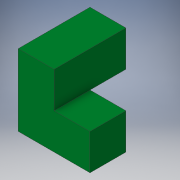
# Autodesk Inventor part: Green part
Saved by Autodesk Inventor 2017 (Build 210142000, 142)
## iProperties
Created: 2016-11-01
Part Number: Green part
Material: Generic
Document SubType Name: Modeling
Designer: rbibb
Density: 1 g/cm^3
Appearance: Default
Author: rbibb
Autodesk Inventor part; units mm, degrees
ref_plane "YZ Plane" through (0, 0, 0) normal (1, 0, 0) x (0, 1, 0)
ref_plane "XZ Plane" through (0, 0, 0) normal (0, 1, 0) x (-1, 0, 0)
ref_plane "XY Plane" through (0, 0, 0) normal (0, 0, 1) x (1, 0, 0)
sketch "Sketch1" plane through (0, 0, 0) normal (1, 0, 0) x (0, 1, 0)
  line L0 (14.195, 33.7604) -> (-4.855, 33.7604)
  line L1 (-4.855, 33.7604) -> (-4.855, -4.3396)
  line L2 (-4.855, -4.3396) -> (14.195, -4.3396)
  line L3 (14.195, -4.3396) -> (14.195, 33.7604)
  point P0 (0, 0)
  dimension "d0" = 19.05
  dimension "d1" = 38.1
  constraints: 8 end point, 2 parallel, 1 horizontal, 1 perpendicular
  measures "d0" distance of L2.end L1.end
  measures "d1" distance of L2.end L0.start
extrude "Extrusion1" add sketch "Sketch1" along normal blind 19.05
sketch "Sketch2" plane through (0, -4.855, -4.3396) normal (0, -1, 0) x (1, 0, 0)
  line L0 (0, 38.1) -> (38.1, 38.1)
  line L1 (38.1, 38.1) -> (38.1, 19.05)
  line L2 (38.1, 19.05) -> (0, 19.05)
  line L3 (0, 19.05) -> (0, 38.1)
  point P0 (0, 4.3396)
  dimension "d4" = 38.1
  dimension "d5" = 19.05
  constraints: 8 end point, 2 parallel, 1 horizontal, 1 perpendicular
  measures "d4" distance of L1.end L2.end
  measures "d5" distance of L0.end L1.end
extrude "Extrusion2" add sketch "Sketch2" along normal blind 19.05
body "Solid1"
